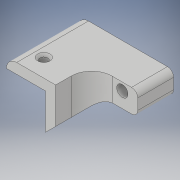
# Autodesk Inventor part: kallax-irja-hook
Saved by Autodesk Inventor 2019.3 (Build 233278000, 278)
## iProperties
Created: 2019-12-14
Part Number: kallax-irja-hook
Material: Generic
Document SubType Name: Modeling
Designer: Frienddo
Density: 1 g/cm^3
Appearance: Default
Author: Frienddo
Autodesk Inventor part; units mm, degrees
ref_plane "YZ Plane" through (0, 0, 0) normal (1, 0, 0) x (0, 1, 0)
ref_plane "XZ Plane" through (0, 0, 0) normal (0, 1, 0) x (-1, 0, 0)
ref_plane "XY Plane" through (0, 0, 0) normal (0, 0, 1) x (1, 0, 0)
sketch "Sketch1" plane through (0, 0, 0) normal (0, 0, 1) x (1, 0, 0)
  line L0 (19, 0) -> (-19, 0)
  arc A0 (-9, 10) -> (-19, 0) centre (-9, 0) ccw
  line L1 (-9, 10) -> (68, 10)
  arc A1 (74, 4) -> (68, 10) centre (68, 4) ccw
  line L2 (74, 4) -> (74, -6.5)
  arc A2 (68, -12.5) -> (74, -6.5) centre (68, -6.5) ccw
  line L3 (68, -12.5) -> (51.8553, -12.5)
  arc A3 (51.8553, -12.5) -> (34.1777, -19.8223) centre (51.8553, -37.5) ccw
  line L4 (34.1777, -19.8223) -> (19, -35)
  line L5 (19, -35) -> (19, 0)
  line L6 (19, 0) -> (19, -22.9675) construction
  circle A4 centre (59, 2.5) radius 5.5
  point P0 (0, 0)
  point P1 (0, 0)
  dimension "d0" = 19
  dimension "d5" = 10
  dimension "d6" = 35
  dimension "d7" = 40
  dimension "d8" = 15
  dimension "d9" = 15
  dimension "d12" = 6
  dimension "d13" = 25
  dimension "d14" = 11
  dimension "d15" = 7.5
  dimension "d30" = 19
  dimension "d31" = 45
  constraints: 14 end point, 8 point on circle, 7 tangent, 5 centre point, 2 horizontal, 2 vertical, 1 coincident, 1 midpoint, 1 parallel, 1 perpendicular, 1 point on line, 1 vertical alignment
  measures "d0" distance of L0.end point (0, 0)
  measures "d5" distance between parallel lines of L1 L0
  measures "d6" distance from line of L4.end L0
  measures "d7" distance from line of L6 A4.centre
  measures "d8" distance from line of L2 A4.centre
  measures "d9" distance from line of L3 A4.centre
  measures "d12" radius of A1
  measures "d13" radius of A3
  measures "d14" diameter of A4
  measures "d15" distance from line of L1 A4.centre
  measures "d30" distance from line of point (0, 0) L5
  measures "d31" angle of L5 L4
extrude "Extrusion1" add sketch "Sketch1" along normal blind 17.5 and the other way blind 52.5
sketch "Sketch3" plane through (-9, 10, 17.5) normal (0, 1, 0) x (1, 0, 0)
  circle A0 centre (9, 17.5) radius 3.75
  circle A1 centre (9, 17.5) radius 6
  dimension "d23" = 7.5
  dimension "d24" = 12
  constraints: 2 centre point, 2 coincident
  measures "d23" diameter of A0
  measures "d24" diameter of A1
extrude "Extrusion3" cut sketch "Sketch3" against normal through all contours A0
chamfer "Chamfer1" distance 2.25 angle 45 1 edges at (-3.75, 10, 0)
sketch "Sketch5" plane through (-9, 10, 17.5) normal (0, 1, 0) x (1, 0, 0)
  line L0 (28, 70) -> (28, 0) projected
  line L1 (83, 70) -> (83, 0) projected
  line L2 (83, 70) -> (83, 0) projected
  line L3 (83, 70) -> (28, 70)
  line L4 (0, 70) -> (77, 70) projected
  line L5 (28, 0) -> (38, 0)
  line L6 (77, 0) -> (0, 0) projected
  line L7 (83, 70) -> (83, 0) projected
  line L8 (83, 35) -> (58, 35)
  arc A0 (58, 35) -> (38, 15) centre (58, 15) ccw
  line L9 (38, 15) -> (38, 0)
  line L10 (38, 0) -> (83, 0)
  point P0 (9, 17.5)
  dimension "d32" = 10
  dimension "d33" = 35
  dimension "d34" = 20
  constraints: 10 end point, 2 point on circle, 2 tangent, 1 centre point, 1 collinear, 1 horizontal, 1 midpoint, 1 perpendicular, 1 point on line, 1 vertical
  measures "d32" distance between parallel lines of L0 L9
  measures "d33" distance between parallel lines of L5 L8
  measures "d34" radius of A0
extrude "Extrusion4" cut sketch "Sketch5" against normal through all contours L9 A0 L8 L1 L10 L6
body "Solid1"
